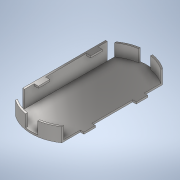
# Autodesk Inventor part: VR_Telefon_Tutucu
Saved by Autodesk Inventor 2022 (Build 260153070, 153G)
## iProperties
Created: 2021-10-26
Part Number: VR_Telefon_Tutucu
Material: Stainless Steel, Austenitic
Document SubType Name: Modeling
Designer: doguh
Density: 8 g/cm^3
Appearance: Semi-Polished
Author: doguh
## iProperties of the stored document VR_Telefon_Tutucu_3DPrint.ipt
Created: 2021-10-26
Part Number: VR_Telefon_Tutucu_3DPrint
Material: Generic
Document SubType Name: Modeling
Designer: doguh
Density: 1 g/cm^3
Appearance: Default
Author: doguh
Autodesk Inventor part; units mm, degrees
ref_plane "YZ Plane" through (0, 0, 0) normal (1, 0, 0) x (0, 1, 0)
ref_plane "XZ Plane" through (0, 0, 0) normal (0, 1, 0) x (-1, 0, 0)
ref_plane "XY Plane" through (0, 0, 0) normal (0, 0, 1) x (1, 0, 0)
sketch "Sketch1" plane through (0, 0, 0) normal (0, 1, 0) x (-1, 0, 0)
  line L0 (38, 68) -> (38, -68)
  line L1 (-38, -68) -> (-38, 68)
  line L2 (-38, 68) -> (38, -68) construction
  line L3 (38, 68) -> (-38, -68) construction
  line L4 (0, -68) -> (0, -80)
  arc A0 (-38, -68) -> (38, -68) centre (0, -13.8333) ccw
  arc A1 (38, 68) -> (-38, 68) centre (0, 13.8333) ccw
  line L5 (38, -68) -> (38, 68)
  line L6 (-38, 68) -> (-38, 53)
  line L7 (-38, -68) -> (-38, -53)
  line L8 (-38, -53) -> (-38, -34)
  line L9 (-38, 53) -> (-38, 34)
  line L10 (38, -68) -> (38, 68)
  line L11 (38, 68) -> (41, 68)
  line L12 (41, 68) -> (41, -68)
  line L13 (41, -68) -> (38, -68)
  line L14 (38, -68) -> (38, 68)
  line L15 (-38, 68) -> (-38, 53)
  line L16 (-38, 34) -> (-38, 53)
  line L17 (-38, -68) -> (-38, -53)
  line L18 (-38, -34) -> (-38, -53)
  line L19 (-38, 68) -> (-38, 52.5)
  line L20 (-38, 52.5) -> (-44, 52.5)
  line L21 (-44, 52.5) -> (-44, 33.5)
  line L22 (-44, 33.5) -> (-38, 33.5)
  line L23 (-38, 33.5) -> (-38, 52.5)
  line L24 (-38, 33.5) -> (-38, -33.5)
  line L25 (-38, -33.5) -> (-44, -33.5)
  line L26 (-44, -33.5) -> (-44, -52.5)
  line L27 (-44, -52.5) -> (-38, -52.5)
  line L28 (-38, -52.5) -> (-38, -33.5)
  point P0 (0, 0)
  dimension "d129" = 3
  constraints: 58 end point, 7 parallel, 6 point on line, 5 point on circle, 3 horizontal, 3 perpendicular, 2 centre point, 2 collinear, 2 midpoint, 1 vertical
  measures "d129" distance of L12.end L13.end
extrude "taban" add sketch "Sketch1" along normal blind 3
sketch "Sketch2" plane through (0, 3, 0) normal (0, 1, 0) x (1, 0, 0)
  line L0 (-41.0189, -68) -> (-38.0189, -68)
  line L1 (-38.0189, -68) -> (-38.0189, 68)
  line L2 (-38.0189, 68) -> (-41.0189, 68)
  line L3 (-41.0189, 68) -> (-41.0189, -68)
  point P0 (0, 0)
  dimension "d45" = 3
  dimension "d46" = 136
  constraints: 8 end point, 2 parallel, 1 horizontal, 1 perpendicular
  measures "d45" distance of L2.end L1.end
  measures "d46" distance of L1.end L0.end
extrude "direk" add sketch "Sketch2" along normal blind 28
sketch "Sketch5" plane through (-38.0189, 3, 68) normal (1, 0, 0) x (0, 0, -1)
  line L0 (15.5, 28) -> (34.5, 28)
  line L1 (34.5, 28) -> (34.5, 25)
  line L2 (34.5, 25) -> (15.5, 25)
  line L3 (15.5, 25) -> (15.5, 28)
  line L4 (101.5, 28) -> (120.5, 28)
  line L5 (120.5, 28) -> (120.5, 25)
  line L6 (120.5, 25) -> (101.5, 25)
  line L7 (101.5, 25) -> (101.5, 28)
  point P0 (68, -3)
  point P1 (0, 28)
  constraints: 16 end point, 4 parallel, 2 horizontal, 2 perpendicular
extrude "sikigecme" add sketch "Sketch5" along normal blind 7
sketch "Sketch6" plane through (0, 3, 0) normal (0, 1, 0) x (1, 0, 0)
  line L0 (-41, -68) -> (-38, -68) projected
  line L1 (-38, -68) -> (-38, -83)
  arc A0 (-38, -68) -> (38, -68) centre (0, -13.8333) ccw projected
  line L2 (38, -68) -> (38, -83)
  arc A1 (-38, -83) -> (38, -83) centre (0, -28.8333) ccw
  arc A2 (38, 68) -> (-38, 68) centre (0, 13.8333) ccw projected
  line L3 (-38, 68) -> (-38, 83)
  line L4 (38, 68) -> (38, 83)
  arc A3 (38, 83) -> (-38, 83) centre (0, 28.8333) ccw
  arc A4 (-38, -68) -> (38, -68) centre (0, -13.8333) ccw
  arc A5 (38, 68) -> (-38, 68) centre (0, 13.8333) ccw
  point P0 (0, 0)
  dimension "d66" = 15
  dimension "d67" = 15
  dimension "d99" = 15
  dimension "d100" = 15
  constraints: 8 end point, 8 point on circle, 4 centre point, 4 vertical
  measures "d66" distance of L3.start L3.end
  measures "d67" distance of L4.start L4.end
  measures "d99" distance of L0.end L1.end
  measures "d100" distance of L2.start L2.end
extrude "fazlalik" add sketch "Sketch6" against normal blind 3
sketch "Sketch7" plane through (0, 3, 0) normal (0, 1, 0) x (1, 0, 0)
  arc A0 (-38, -83) -> (38, -83) centre (0, -28.8333) ccw projected
  line L0 (-38, -83) -> (-38, -80)
  line L1 (38, -83) -> (38, -80)
  arc A1 (-38, -80) -> (38, -80) centre (0, -25.8333) ccw
  arc A2 (-38, -83) -> (38, -83) centre (0, -28.8333) ccw
  arc A3 (38, 83) -> (-38, 83) centre (0, 28.8333) ccw projected
  line L2 (-38, 83) -> (-38, 80)
  line L3 (-38, 68) -> (-38, 83) projected
  line L4 (38, 52.5) -> (38, 83) projected
  line L5 (38, 83) -> (38, 80)
  arc A4 (38, 80) -> (-38, 80) centre (0, 25.8333) ccw
  arc A5 (38, 83) -> (-38, 83) centre (0, 28.8333) ccw
  point P0 (0, 0)
  point P1 (38, 53)
  point P2 (38, -34)
  dimension "d74" = 3
  dimension "d75" = 3
  dimension "d102" = 3
  dimension "d103" = 3
  constraints: 8 end point, 8 point on circle, 4 centre point, 2 point on line, 1 concentric
  measures "d74" distance of L2.start L2.end
  measures "d75" distance of L4.end L5.end
  measures "d102" distance of L1.start L1.end
  measures "d103" distance of L0.start L0.end
extrude "yandirek" add sketch "Sketch7" along normal blind 20
sketch "Sketch9" plane through (0, 3, 0) normal (0, 1, 0) x (1, 0, 0)
  arc A0 (-38, -83) -> (38, -83) centre (0, -28.8333) ccw projected
  line L0 (-10, -94.24) -> (-10, -91.24)
  arc A1 (-38, -80) -> (38, -80) centre (0, -25.8333) ccw projected
  line L1 (10, -94.24) -> (10, -91.24)
  arc A2 (-10, -94.24) -> (10, -94.24) centre (0, -28.8333) ccw
  arc A3 (-10, -91.24) -> (10, -91.24) centre (0, -25.8333) ccw
  arc A4 (38, 83) -> (-38, 83) centre (0, 28.8333) ccw projected
  line L2 (10.1599, 94.2153) -> (10, 91.24)
  arc A5 (38, 80) -> (-38, 80) centre (0, 25.8333) ccw projected
  line L3 (-10, 94.24) -> (-10, 91.24)
  arc A6 (10, 91.24) -> (-10, 91.24) centre (0, 25.8333) ccw
  arc A7 (10.1599, 94.2153) -> (-10, 94.24) centre (0, 28.8333) ccw
  point P0 (0, 0)
  point P1 (10, -91.24)
  point P2 (-10, 94.24)
  constraints: 14 point on circle, 8 end point, 4 centre point
extrude "yanbosluk" cut sketch "Sketch9" along normal blind 20
body "Solid1"
